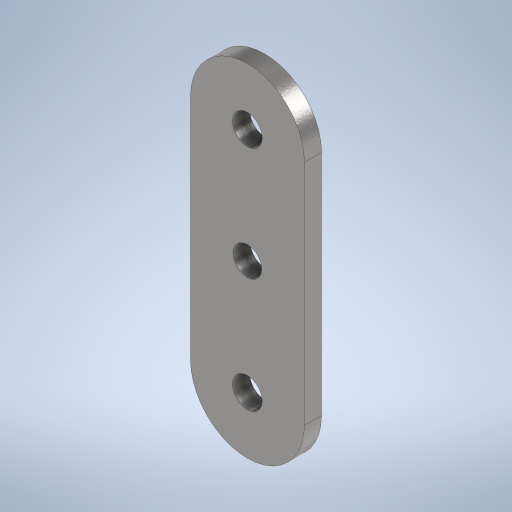
# Autodesk Inventor part: FingerSupport
Saved by Autodesk Inventor 2024.2 (Build 282272000, 272)
## iProperties
Created: 2025-04-11
Part Number: FingerSupport
Material: Generic
Document SubType Name: Modeling
Designer: Admin
Density: 1 g/cm^3
Appearance: Knurled 45
Author: Admin
Autodesk Inventor part; units mm, degrees
ref_plane "YZ Plane" through (0, 0, 0) normal (1, 0, 0) x (0, 1, 0)
ref_plane "XZ Plane" through (0, 0, 0) normal (0, 1, 0) x (-1, 0, 0)
ref_plane "XY Plane" through (0, 0, 0) normal (0, 0, 1) x (1, 0, 0)
sketch "Sketch1" plane through (0, 0, 0) normal (0, 0, 1) x (1, 0, 0)
  line L0 (0, 0) -> (0, 20) construction
  line L1 (0, 0) -> (0, 20) construction
  line L2 (0, 20) -> (0, -20) construction
  line L3 (-10, 20) -> (-10, -20)
  line L4 (10, -20) -> (10, 20)
  arc A0 (10, 20) -> (-10, 20) centre (0, 20) ccw
  arc A1 (-10, -20) -> (10, -20) centre (0, -20) ccw
  circle A2 centre (0, 20) radius 2.6
  line L5 (0, 0) -> (10, 0) construction
  circle A3 centre (0, -20) radius 2.6
  circle A4 centre (0, 0) radius 2.5
  dimension "d15" = 20
  dimension "d16" = 20
  dimension "d17" = 40
  dimension "d18" = 10
  dimension "d19" = 5.2
  dimension "d20" = 5
  constraints: 14 end point, 5 centre point, 4 point on circle, 4 tangent, 2 coincident, 2 midpoint, 2 vertical, 1 parallel, 1 point on line, 1 symmetric about line, 1 other
  measures "d15" distance of L0.start L0.end
  measures "d16" distance of L0.start L1.end
  measures "d17" distance of L1.end L2.end
  measures "d18" distance between parallel lines of L4 L2
  measures "d19" diameter of A2
  measures "d20" diameter of A4
extrude "Extrusion1" add sketch "Sketch1" along normal blind 3
body "Solid1"
